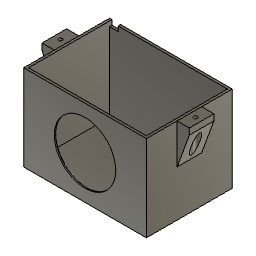
earrestroyer-case (Autodesk Fusion 360 design; units mm, degrees)
Autodesk Fusion 360 part; units mm, degrees
note: some values were not read from the file. Set by a fixed rule: which face or edge a step refers to.
sketch "Base" plane through (0, 0, 0) normal (0, 0, 1) x (1, 0, 0) in component "Case"
  line L0 (0, 0) -> (100, 0)
  line L1 (100, 0) -> (100, 70)
  line L2 (100, 70) -> (0, 70)
  line L3 (0, 70) -> (0, 0)
  line L4 (100, 27.5453) -> (100, 47.5453)
  line L5 (0, 35) -> (100, 35) construction
  line L6 (50, 70) -> (50, 0) construction
  dimension "d1" = 100
  dimension "d2" = 70
  constraint horizontal L0
  constraint vertical L1
  constraint horizontal L2
  constraint vertical L3
  constraint coincident L0.start L3.end
  constraint vertical L4
  constraint coincident L1 L4.end
  constraint midpoint L3 L5.start
  constraint midpoint L1 L5.end
  constraint midpoint L2 L6.start
  constraint midpoint L0 L6.end
  measures "d1" distance of L0.start L0.end
  measures "d2" distance of L0.start L2.end
extrude "Extrude3" add sketch "Base" along normal blind 70 makes body 1 in component "Case"
shell "Shell2" thickness 2 removed faces 1 at (33.3333, 32.5151, 70) on bodies 1 in component "Case"
ref_plane "WorkPlane5" through (50, 35, 36) normal (1, 0, 0) x (0, 1, 0) in component "Case"
ref_plane "WorkPlane6" through (50, 35, 36) normal (0, 0, 1) x (1, 0, 0) in component "Case"
sketch "Sketch10" plane through (50, 35, 36) normal (0, 0, 1) x (1, 0, 0) in component "Case"
sketch "Sketch11" plane through (0, 0, 0) normal (0, 1, 0) x (1, 0, 0) in component "Case"
ref_plane "WorkPlane7" through (50, 35, 36) normal (0, -1, 0) x (1, 0, 0) in component "Case"
sketch "Sketch12" plane through (50, 35, 36) normal (0, -1, 0) x (1, 0, 0) in component "Case"
  line L0 (-60, 34) -> (-60, 29)
  line L1 (-60, 29) -> (-50, 1.5252)
  line L2 (-50, 1.5252) -> (-50, 34)
  line L3 (-50, 34) -> (-60, 34)
  point P0 (-48, 34)
  dimension "d100" = 5
  dimension "d101" = 10
  dimension "d102" = 20
  constraint vertical L0
  constraint parallel L0 L2
  constraint perpendicular L2 L3
  constraint coincident L3 P0
  measures "d100" distance of L0.start L0.end
  measures "d101" distance of L0.start L2.end
  measures "d102" angle of L1 L2
extrude "Extrude9" add sketch "Sketch12" along normal mid plane 20 separate body makes body 2 in component "Case"
sketch "Sketch1" plane through (0, 0, 0) normal (0, -1, 0) x (1, 0, 0)
  line L0 (0, 0) -> (100, 0)
  line L1 (100, 0) -> (100, 70)
  line L2 (100, 70) -> (0, 70)
  line L3 (0, 70) -> (0, 0)
  circle A0 centre (50, 35) radius 25
  dimension "d47" = 50
  dimension "d48" = 50
  dimension "d49" = 35
  measures "d47" diameter of A0
  measures "d48" distance of L1 A0.centre
  measures "d49" distance of L2 A0.centre
ref_plane "WorkPlane8" through (-5, 35, 70) normal (0, 0, 1) x (-1, 0, 0) in component "Case"
sketch "Sketch13" plane through (-5, 35, 70) normal (0, 0, 1) x (1, 0, 0) in component "Case"
  circle A0 centre (0, 0) radius 1.5
  dimension "d94" = 3
  constraint coincident A0.centre origin
  measures "d94" diameter of A0
extrude "Extrude10" cut sketch "Sketch13" along normal up to surface end surface through (-10, 35, 65) normal (-0.939693, 0, -0.34202) offset 0 bodies 2 in component "Case"
ref_plane "WorkPlane12" through (-5, 35, 37.5252) normal (0, 0, 1) x (-1, 0, 0) in component "Case"
sketch "Sketch17" plane through (-5, 35, 37.5252) normal (0, 0, 1) x (1, 0, 0) in component "Case"
  circle A0 centre (0, 0) radius 3.5
  dimension "d106" = 7
  constraint coincident A0.centre origin
  measures "d106" diameter of A0
extrude "Extrude11" cut sketch "Sketch17" along normal up to surface (27.4748 mm away) bodies 2 in component "Case"
extrude "Extrude5" cut sketch "Sketch1" against normal up to surface (2 mm away) contours A0 bodies 1 in component "Case"
sketch "Led" plane through (0, 0, 2) normal (0, 0, 1) x (-1, 0, 0) in component "Case"
  line L0 (-98, -2) -> (-98, -68)
  line L1 (-98, -68) -> (-2, -68)
  line L2 (-2, -68) -> (-2, -2)
  line L3 (-2, -2) -> (-98, -2)
  line L4 (-4, -9) -> (-6, -9)
  line L5 (-6, -9) -> (-6, -4)
  line L6 (-6, -4) -> (-4, -4)
  line L7 (-4, -4) -> (-4, -9)
  line L8 (0, 0) -> (-100, 0)
  line L9 (0, -70) -> (0, 0)
  dimension "d52" = 2
  dimension "d53" = 5
  dimension "d68" = 4
  dimension "d69" = 4
  constraint horizontal L4
  constraint vertical L5
  constraint horizontal L6
  constraint vertical L7
  measures "d52" distance of L4.start L4.end
  measures "d53" distance of L4.start L6.end
  measures "d68" distance of L6.end L8
  measures "d69" distance of L7 L9
extrude "Extrude6" cut sketch "Led" against normal up to surface (2 mm away) contours L4 L5 L6 L7 bodies 1 in component "Case"
sketch "Text" plane through (0, 0, 0) normal (0, 0, -1) x (1, 0, 0) in component "Case"
  line L0 (6, -4) -> (6, -9)
  line L1 (6, -9) -> (4, -9)
  line L2 (4, -9) -> (4, -4)
  line L3 (4, -4) -> (6, -4)
  line L4 (100, -70) -> (100, 0)
  line L5 (100, 0) -> (0, 0)
  line L6 (0, 0) -> (0, -70)
  line L7 (0, -70) -> (100, -70)
  line L8 (6.8891, -81.127) -> (89.8891, -81.127) construction
  line L9 (89.8891, -81.127) -> (89.8891, -27.127) construction
  line L10 (89.8891, -27.127) -> (6.8891, -27.127) construction
  line L11 (6.8891, -27.127) -> (6.8891, -81.127) construction
  dimension "d58" = 10
  text T0 "EarDestroyer" font "Verdana" height 10 align left top in box 83 x 54 at (6.8891, -81.127) x (1, 0) y (0, 1) spacing 1
sketch "Gate" plane through (0, 70, 0) normal (0, 1, 0) x (-1, 0, 0) in component "Case"
  line L0 (-100, 0) -> (0, 0)
  line L1 (0, 70) -> (-100, 70)
  line L2 (-100, 70) -> (-100, 0)
  line L3 (-2, 66.007) -> (-9, 66.007)
  line L4 (-9, 66.007) -> (-9, 70.007)
  line L5 (-9, 70.007) -> (-2, 70.007)
  line L6 (-2, 70.007) -> (-2, 66.007)
  line L7 (0, 70) -> (-100, 70)
  line L8 (-100, 70) -> (-100, 0)
  line L9 (-100, 0) -> (0, 0)
  line L10 (0, 0) -> (0, 70)
  line L11 (0, 37.5252) -> (0, 70)
  dimension "d61" = 7
  dimension "d91" = 4
  dimension "d92" = 2
  constraint horizontal L3
  constraint vertical L4
  constraint horizontal L5
  constraint vertical L6
  constraint horizontal L7
  constraint vertical L8
  constraint horizontal L9
  constraint vertical L10
  constraint coincident L0.start L2.end
  constraint coincident L1.start L7.start
  measures "d61" distance of L3.start L3.end
  measures "d91" distance of L3.end L4.end
  measures "d92" distance of L6 L11
extrude "Extrude8" cut sketch "Gate" against normal up to surface (2 mm away) contours L1 L4 L5 L6 L7 | L1 L3 L4 L6 L7 bodies 1 in component "Case"
extrude "Extrude7" cut sketch "Text" against normal blind 1 text T0 bodies 1 in component "Case"
fillet "Fillet2" radius 1 1 edges at (26.6918, 2, 25.9596) on bodies 1 in component "Case"
mirror "Mirror4" about plane through (50, 35, 36) normal (1, 0, 0) of bodies 2 makes body 3 in component "Case"
component "Case" placed x (1, 0, 0) y (0, 1, 0) z (0, 0, 1) at (0, 0, 0)
named bodies: "Box", "ScrewHoleL", "ScrewHoleR"
